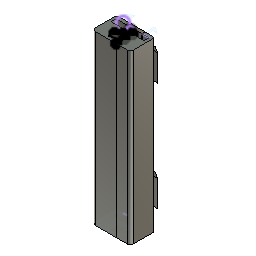
Clip_Lamps_Pixel_x2Leds (Autodesk Fusion 360 design; units mm, degrees)
Autodesk Fusion 360 part; units mm, degrees
note: some values were not read from the file. Chosen so that the rebuilt part matches the saved one: which bodies a step acts on; which face or edge a step refers to. Set by a fixed rule: which sketch regions a step uses.
sketch "Esquisse1" plane through (0, 0, 0) normal (0, 0, 1) x (-1, 0, 0)
  line L0 (2.9, -0.75) -> (2.9, -4.25)
  arc A0 (2.9, -4.25) -> (3.2087, -4.4179) centre (3.1, -4.25) ccw
  line L1 (3.2087, -4.4179) -> (5.2, -3.1288)
  line L2 (5.2, -3.1288) -> (3.7, -3.1288)
  line L3 (3.7, -3.1288) -> (3.7, -1.7288)
  arc A1 (3.7, -1.7288) -> (5.6201, -1.5684) centre (0, 54.1488) ccw
  arc A2 (5.6201, -1.5684) -> (5.8, -1.3695) centre (5.6, -1.3695) ccw
  line L4 (5.8, -1.3695) -> (5.8, 4.75)
  arc A3 (5.8, 4.75) -> (4.8, 5.75) centre (4.8, 4.75) ccw
  line L5 (4.8, 5.75) -> (-4.8, 5.75)
  arc A4 (-4.8, 5.75) -> (-5.8, 4.75) centre (-4.8, 4.75) ccw
  line L6 (-5.8, 4.75) -> (-5.8, -1.3695)
  arc A5 (-5.8, -1.3695) -> (-5.6201, -1.5684) centre (-5.6, -1.3695) ccw
  arc A6 (-5.6201, -1.5684) -> (-3.7, -1.7288) centre (0, 54.1488) ccw
  line L7 (-3.7, -1.7288) -> (-3.7, -3.1288)
  line L8 (-3.7, -3.1288) -> (-5.2, -3.1288)
  line L9 (-5.2, -3.1288) -> (-3.2087, -4.4179)
  arc A7 (-3.2087, -4.4179) -> (-2.9, -4.25) centre (-3.1, -4.25) ccw
  line L10 (-2.9, -4.25) -> (-2.9, -0.75)
  line L11 (-2.9, -0.75) -> (-5, -0.75)
  line L12 (-5, -0.75) -> (-5, 0.75)
  line L13 (-5, 0.75) -> (5, 0.75)
  line L14 (5, 0.75) -> (5, -0.75)
  line L15 (5, -0.75) -> (2.9, -0.75)
  point P0 (0, 0.75)
  point P1 (5, 0)
  dimension "d1" = 10
  dimension "d2" = 1.5
  dimension "d3" = 7.4
  dimension "d4" = 0.8
  dimension "d5" = 0.8
  dimension "d6" = 5
  dimension "d7" = 1
  dimension "d8" = 0.2
  dimension "d9" = 56
  dimension "d13" = 0.9788
  dimension "d14" = 0.8184
  dimension "d15" = 1.5
  dimension "d16" = 1.4
  dimension "d18" = 0.2
  dimension "d19" = 3.5
  dimension "d48" = 11.6
  constraint horizontal L13
  constraint vertical L14
  constraint horizontal L15
  constraint vertical L0
  constraint vertical L10
  constraint horizontal L11
  constraint vertical L7
  constraint vertical L6
  constraint horizontal L5
  constraint vertical L4
  constraint horizontal L2
  constraint horizontal L8
  constraint equal L0 L10
  constraint equal L11 L15
  constraint equal L12 L14
  constraint equal L4 L6
  constraint equal L3 L7
  constraint equal L2 L8
  constraint vertical L3
  constraint midpoint L13 P0
  constraint midpoint L14 P1
  constraint horizontal origin P1
  constraint vertical origin P0
  constraint tangent A2 L4
  constraint tangent A1 A2
  constraint vertical origin A1.centre
  constraint tangent A3 L5
  constraint tangent L4 A3
  constraint tangent L5 A4
  constraint tangent A4 L6
  constraint tangent L6 A5
  constraint tangent A5 A6
  constraint equal A3 A4
  constraint horizontal A1.end A5.end
  constraint horizontal L3.end A6.end
  constraint tangent L0 A0
  constraint tangent A0 L1
  constraint tangent A7 L10
  constraint tangent L9 A7
  constraint equal L1 L9
  constraint equal A0 A7
  measures "d1" distance of L12.end L13.end
  measures "d2" distance of L13.end L14.end
  measures "d3" distance of L3 L7
  measures "d4" distance of L0 L3
  measures "d5" distance of L4 L14
  measures "d6" distance of L5 L13
  measures "d7" radius of A3
  measures "d8" radius of A2
  measures "d9" radius of A1
  measures "d13" distance of L3.end L15
  measures "d14" distance of A1.end L15
  measures "d15" distance of L1.end L2.end
  measures "d16" distance of L2.end L3.end
  measures "d18" radius of A0
  measures "d19" distance of L0.start L0.end
  measures "d48" distance of L4 L6
extrude "Extrusion1" add sketch "Esquisse1" along normal blind 51 makes body 1
sketch "Esquisse2" plane through (0, 0, 51) normal (0, 0, 1) x (-1, 0, 0)
  line L0 (5, -0.75) -> (2.9, -0.75)
  line L1 (2.9, -0.75) -> (2.9, -4.25)
  arc A0 (2.9, -4.25) -> (3.2087, -4.4179) centre (3.1, -4.25) ccw
  line L2 (3.2087, -4.4179) -> (5.2, -3.1288)
  line L3 (5.2, -3.1288) -> (3.7, -3.1288)
  line L4 (3.7, -3.1288) -> (3.7, -1.7288)
  arc A1 (3.7, -1.7288) -> (5.6201, -1.5684) centre (0, 54.1488) ccw
  arc A2 (5.6201, -1.5684) -> (5.8, -1.3695) centre (5.6, -1.3695) ccw
  line L5 (5.8, -1.3695) -> (5.8, 4.75)
  arc A3 (5.8, 4.75) -> (4.8, 5.75) centre (4.8, 4.75) ccw
  line L6 (4.8, 5.75) -> (-4.8, 5.75)
  arc A4 (-4.8, 5.75) -> (-5.8, 4.75) centre (-4.8, 4.75) ccw
  line L7 (-5.8, 4.75) -> (-5.8, -1.3695)
  arc A5 (-5.8, -1.3695) -> (-5.6201, -1.5684) centre (-5.6, -1.3695) ccw
  arc A6 (-5.6201, -1.5684) -> (-3.7, -1.7288) centre (0, 54.1488) ccw
  line L8 (-3.7, -1.7288) -> (-3.7, -3.1288)
  line L9 (-3.7, -3.1288) -> (-5.2, -3.1288)
  line L10 (-5.2, -3.1288) -> (-3.2087, -4.4179)
  arc A7 (-3.2087, -4.4179) -> (-2.9, -4.25) centre (-3.1, -4.25) ccw
  line L11 (-2.9, -4.25) -> (-2.9, -0.75)
  line L12 (-5, -0.75) -> (-5, 0.75)
  line L13 (-5, 0.75) -> (5, 0.75)
  line L14 (5, 0.75) -> (5, -0.75)
  line L15 (-1.5, 0.75) -> (-1.5, 2.5)
  line L16 (-1.5, 2.5) -> (1.5, 1.75)
  line L17 (1.5, 1.75) -> (1.5, 4.75)
  line L18 (1.5, 4.75) -> (-1.5, 4)
  line L19 (-1.5, 4) -> (-1.5, 5.75)
  line L20 (-1.5, 4) -> (-1.5, 2.5) construction
  line L21 (-2.9, -0.75) -> (-5, -0.75)
  point P0 (-1.5, 3.25)
  point P1 (1.5, 3.25)
  point P2 (0, 2.125)
  dimension "d22" = 3
  dimension "d23" = 1.5
  dimension "d24" = 3
  constraint coincident L13 L15.start
  constraint perpendicular L13 L15
  constraint perpendicular L13 L17
  constraint coincident L6 L19.end
  constraint perpendicular L6 L19
  constraint equal L15 L19
  constraint vertical L15.end L18.end
  constraint midpoint L20 P0
  constraint midpoint L17 P1
  constraint horizontal P0 P1
  constraint midpoint L16 P2
  constraint vertical origin P2
  measures "d22" distance of L15 L17
  measures "d23" distance of L15.end L18.end
  measures "d24" distance of L16.end L17.end
split "Scinder1" by curves path "Esquisse2" along L15 L16 L17 L18 L19 bodies 1 makes body 2 at (-2.8333, -0.75, 34)
move_face "DécalerLesFaces1" offset -0.2 3 faces at (0.5, -2.25, 17) (-1.5, -2.75, 34) (-0.5, -4.5, 17) on bodies 2
sketch "Esquisse3" plane through (3.7, 0, 0) normal (1, 0, 0) x (0, 1, 0)
  line L0 (1.7288, 0) -> (3.1288, 0)
  line L1 (3.1288, 0) -> (3.1288, 51)
  line L2 (3.1288, 51) -> (1.7288, 51)
  line L3 (1.7288, 51) -> (1.7288, 0)
  line L4 (1.7288, 38) -> (1.7288, 13)
  line L5 (1.7288, 38) -> (6.7288, 38)
  line L6 (6.7288, 38) -> (6.7288, 13)
  line L7 (6.7288, 13) -> (1.7288, 13)
  dimension "d30" = 5
  dimension "d31" = 13
  dimension "d32" = 25
  constraint vertical L4
  constraint coincident L3 L4.end
  constraint perpendicular L1 L5
  constraint perpendicular L5 L6
  constraint horizontal L7
  measures "d30" distance of L4.end L6.end
  measures "d31" distance of L0 L7
  measures "d32" distance of L5.end L6.end
extrude "Extrusion2" cut sketch "Esquisse3" along normal through all and the other way through all contours L1 L3 L4 L5 L7 | L1 L5 L6 L7 bodies 1 2
sketch "Esquisse7" plane through (3.7, 0, 0) normal (1, 0, 0) x (0, 1, 0)
  line L0 (3.1288, 13) -> (1.7288, 13)
  line L1 (1.7288, 0) -> (4.5288, 0)
  line L2 (4.5288, 0) -> (4.5288, 5)
  line L3 (4.5288, 5) -> (1.7288, 5)
  line L4 (1.7288, 5) -> (1.7288, 0)
  line L5 (1.7288, 51) -> (4.5288, 51)
  line L6 (4.5288, 51) -> (4.5288, 46)
  line L7 (4.5288, 46) -> (1.7288, 46)
  line L8 (1.7288, 46) -> (1.7288, 51)
  point P0 (1.7288, 0)
  point P1 (1.7288, 51)
  dimension "d51" = 2.8
  dimension "d52" = 5
  constraint horizontal L1
  constraint vertical L2
  constraint horizontal L3
  constraint vertical L4
  constraint coincident P0 L1.start
  constraint horizontal L5
  constraint vertical L6
  constraint horizontal L7
  constraint vertical L8
  constraint coincident P1 L5.start
  constraint vertical L2.end L6.end
  constraint equal L2 L6
  measures "d51" distance of P0 L1.end
  measures "d52" distance of L1.end L2.end
extrude "Extrusion5" cut sketch "Esquisse7" against normal through all and the other way through all bodies 1 2
pattern_linear "Réseau R1" count 3 spacing 33 along (0, 0, 1) of "Extrusion2"
sketch "Esquisse4" plane through (0, 0, 0) normal (0, 0, -1) x (1, 0, 0)
  line L0 (1.5, 4.2062) -> (1.5, 5.75)
  line L1 (1.5, 5.75) -> (-4.8, 5.75)
  arc A0 (-4.8, 5.75) -> (-5.8, 4.75) centre (-4.8, 4.75) ccw
  line L2 (-5.8, 4.75) -> (-5.8, -1.3695)
  arc A1 (-5.8, -1.3695) -> (-5.6201, -1.5684) centre (-5.6, -1.3695) ccw
  arc A2 (-5.6201, -1.5684) -> (-3.7, -1.7288) centre (0, 54.1488) ccw
  line L3 (-2.9, -1.7288) -> (-2.9, -0.75)
  line L4 (-2.9, -0.75) -> (-5, -0.75)
  line L5 (-5, -0.75) -> (-5, 0.75)
  line L6 (-5, 0.75) -> (1.5, 0.75)
  line L7 (1.5, 0.75) -> (1.5, 2.2938)
  line L8 (1.5, 2.2938) -> (-1.7, 1.4938)
  line L9 (-1.7, 1.4938) -> (-1.7, 5.0062)
  line L10 (-1.7, 5.0062) -> (1.5, 4.2062)
  line L11 (-3.7, -1.7288) -> (-2.9, -1.7288)
sketch "Esquisse5" plane through (-2.9, 0, 0) normal (1, 0, 0) x (0, 1, 0)
  line L0 (1.7288, 51) -> (0.75, 51)
  line L1 (0.75, 51) -> (0.75, 0)
  line L2 (0.75, 0) -> (1.7288, 0)
  line L3 (4.25, 13) -> (1.7288, 13)
  line L4 (1.7288, 13) -> (1.7288, 38)
  line L5 (1.7288, 38) -> (4.25, 38)
  line L6 (4.25, 38) -> (4.25, 46)
  line L7 (0.75, 51) -> (1.7288, 51)
  line L8 (1.7288, 51) -> (1.7288, 0)
  line L9 (1.7288, 0) -> (0.75, 0)
  line L10 (0.75, 0) -> (0.75, 51)
  line L11 (1.7288, 0) -> (1.7288, 5)
  line L12 (1.7288, 5) -> (4.25, 5)
  line L13 (4.25, 5) -> (4.25, 13)
  line L14 (4.25, 46) -> (1.7288, 46)
  line L15 (1.7288, 46) -> (1.7288, 51)
  constraint horizontal L7
  constraint vertical L8
  constraint horizontal L9
  constraint vertical L10
  constraint coincident L2 L8.end
  constraint coincident L0.end L1.start
  constraint vertical L3.end L2.end
extrude "Extrusion3" add sketch "Esquisse5" along normal blind 5.7 contours L0 L1 L2 L4 L7 L8 L9 L10 L11 L15 bodies 2
sketch "Esquisse6" plane through (0, 1.7288, 0) normal (0, 1, 0) x (-1, 0, 0)
  line L0 (3.7, 51) -> (-2.8, 51)
  line L1 (-2.8, 51) -> (-2.8, 0)
  line L2 (-2.8, 0) -> (3.7, 0)
  line L3 (2.9, 13) -> (3.7, 13)
  line L4 (3.7, 13) -> (3.7, 38)
  line L5 (3.7, 38) -> (2.9, 38)
  line L6 (2.85, 6.35) -> (-2.85, 6.35)
  line L7 (-2.85, 6.35) -> (-2.85, 11.65)
  line L8 (-2.85, 11.65) -> (2.85, 11.65)
  line L9 (2.85, 11.65) -> (2.85, 6.35)
  line L10 (2.85, 6.35) -> (-2.85, 11.65) construction
  line L11 (-2.85, 6.35) -> (2.85, 11.65) construction
  line L12 (-2.9, 5) -> (-2.9, 13)
  line L13 (2.9, 38) -> (2.9, 46)
  line L14 (2.9, 46) -> (3.7, 46)
  line L15 (3.7, 46) -> (3.7, 51)
  point P0 (0, 9)
  point P1 (-2.9, 9)
  dimension "d40" = 5.7
  dimension "d41" = 5.3
  constraint horizontal L6
  constraint perpendicular L6 L7
  constraint parallel L6 L8
  constraint parallel L7 L9
  constraint coincident L10 P0
  constraint coincident L11 P0
  constraint vertical origin P0
  constraint midpoint L12 P1
  constraint horizontal P0 P1
  measures "d40" distance of L6.start L6.end
  measures "d41" distance of L6.start L8.end
extrude "Extrusion4" cut sketch "Esquisse6" against normal blind 1 bodies 2
pattern_linear "Réseau R2" count 4 spacing 33 along (0, 0, 1) of "Extrusion4"
equation "d20 = 117 mm - 66 mm"
equation "d31 = 8 mm + 5 mm"
named bodies: "Clip Led 2", "Clip Led 1"
